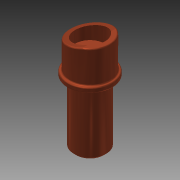
# Autodesk Inventor part: anode-copper
Saved by Autodesk Inventor 2015 (Build 190159000, 159)
## iProperties
Created: 2014-09-24
Part Number: anode-copper
Material: Copper
Document SubType Name: Modeling
Designer: Adam
Density: 8.94 g/cm^3
Appearance: Copper - Satin
Author: Adam
Autodesk Inventor part; units mm, degrees
sketch "Sketch1" plane through (0, 0, 0) normal (0, 0, 1) x (1, 0, 0)
  line L0 (-9.5, 5) -> (-9.5, 21) construction
  line L1 (-8.5, 21) -> (-8.5, 5) construction
  line L2 (-8.5, 5) -> (-9.5, 5) construction
  line L3 (9.5, 21) -> (9.5, 5) construction
  line L4 (9.5, 5) -> (8.5, 5) construction
  line L5 (8.5, 5) -> (8.5, 21) construction
  line L6 (0, -8.3344) -> (0, 50.0061) construction
  line L7 (-39.1105, 0) -> (33.5256, 0) construction
  line L8 (0, 0) -> (-6.5, 0)
  line L9 (-6.5, 0) -> (-6.5, 24)
  line L10 (-6.5, 24) -> (-6, 24)
  line L11 (0, 23) -> (0, 0)
  line L12 (23.149, 37.2995) -> (-28.7339, 37.2995) construction
  line L13 (12.5697, 41.6718) -> (-8, 37.2995) construction
  line L14 (-6, 25) -> (-8, 25)
  line L15 (-8, 27) -> (-8, 37.2995)
  line L16 (-8, 37.2995) -> (-6, 37.2995)
  line L17 (0, 33) -> (0, 24)
  line L18 (0, 24) -> (0, 23)
  line L19 (-6, 25) -> (-6, 24)
  line L20 (0, 33) -> (-6, 33)
  line L21 (-6, 33) -> (-6, 37.2995)
  line L22 (-23.2556, 39) -> (9.8667, 39) construction
  line L23 (-9.5, 6) -> (-9.5, 22) construction
  arc A0 (-6.5, 25) -> (-9.5, 22) centre (-6.5, 22) ccw construction
  line L24 (-6.5, 25) -> (-6, 25) construction
  line L25 (-8.5, 6) -> (-9.5, 6) construction
  line L26 (9.5, 6) -> (8.5, 6) construction
  arc A1 (-6.5, 24) -> (-8.5, 22) centre (-6.5, 22) ccw construction
  line L27 (-6.5, 24) -> (-4.2639, 24) construction
  line L28 (-8, 25) -> (-9, 25)
  line L29 (-9, 25) -> (-9, 27)
  line L30 (-9, 27) -> (-8, 27)
  point P0 (0, 39)
  dimension "d0" = 6.5
  dimension "d2" = 12
  dimension "d3" = 8
  dimension "d4" = 2
  dimension "d5" = 8
  dimension "d10" = 39
  dimension "d26" = 2
  dimension "d27" = 1
  constraints: 58 end point, 10 horizontal, 7 parallel, 6 point on line, 5 vertical, 4 point on circle, 3 perpendicular, 2 centre point, 2 collinear, 19 other
  measures "d0" distance between parallel lines of L6 L9
  measures "d2" angle of L12 L13
  measures "d3" distance between parallel lines of L17 L15
  measures "d4" distance between parallel lines of L15 L21
  measures "d5" distance between parallel lines of L14 L20
  measures "d10" distance between parallel lines of L7 L22
  measures "d26" distance between parallel lines of L28 L30
  measures "d27" distance between parallel lines of L15 L29
revolve "Revolution1" add sketch "Sketch1" angle 360 about axis through (0, 23, 0) along (0, -1, 0)
chamfer "Chamfer1" distance 1 angle 45 1 edges at (6.5, 0, 0)
sketch "Sketch5" plane through (0, 37.2995, 0) normal (0, 1, 0) x (1, 0, 0)
  circle A0 centre (0, 0) radius 8 projected
  circle A1 centre (0, 0) radius 6 projected
  point P0 (0, 0)
ref_plane "Work Plane1" through (0, 0, 3) normal (0, 0, 1) x (1, 0, 0)
sketch "Sketch6" plane through (0, 0, 3) normal (0, 0, 1) x (1, 0, 0)
  line L0 (12.5697, 41.6718) -> (-8, 37.2995) construction
  point P0 (0, 0)
ref_plane "Work Plane2" through (12.5697, 41.6718, 3) normal (0.2079117, -0.9781476, 0) x (-0.9781476, -0.2079117, 0)
extrude "Extrusion1" add sketch "Sketch5" along normal up to surface surface through (12.5697, 41.6718, 3) normal (0.2079117, -0.9781476, 0)
sketch "Sketch7" plane through (0, 0, 0) normal (0, -1, 0) x (1, 0, 0)
  point P0 (0, 0)
  point P1 (0, 0)
  constraints: 1 coincident
hole "Hole1" at (0, 0, 0) direction (0, 1, 0) diameter 6 depth 12 tip angle 118
thread "Thread1" size "1/4-20 UNC" class "2B" standard "ANSI Unified Screw Threads" full length
chamfer "Chamfer2" distance 1 angle 45 1 edges at (0, 0, 3)
fillet "Fillet1" radius 0.5 3 edges at (8, 27, 0) (9, 27, 0) (9, 25, 0)
ref_plane "Work Plane3" through (0, 39.8, 0) normal (0, 1, 0) x (1, 0, 0)
sketch "Sketch8" plane through (0, 39.8, 0) normal (0, 1, 0) x (1, 0, 0)
  circle A0 centre (0, 0) radius 9
  point P0 (0, 0)
  dimension "d30" = 18
  constraints: 1 centre point, 1 coincident
  measures "d30" diameter of A0
extrude "Extrusion2" cut sketch "Sketch8" along normal through all
fillet "Fillet2" radius 0.5 4 edges at (-4.1165, 38.125, -6.8597) (-4.1165, 38.125, 6.8597) (6.8597, 39.8, -4.1165) (6.8597, 39.8, 4.1165)
fillet "Fillet2" radius 1 2 edges at (3.7637, 39.8, 5.8661) (3.7637, 39.8, -5.8661)
body "Solid1"
